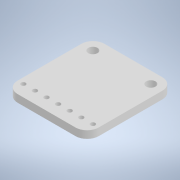
# Autodesk Inventor part: BMP280 footprint
Saved by Autodesk Inventor 2020 (Build 240168000, 168)
## iProperties
Created: 2020-09-26
Part Number: BMP280 footprint
Material: Generic
Document SubType Name: Modeling
Designer: mulve
Density: 1 g/cm^3
Appearance: Default
Author: mulve
Autodesk Inventor part; units mm, degrees
ref_plane "YZ Plane" through (0, 0, 0) normal (1, 0, 0) x (0, 1, 0)
ref_plane "XZ Plane" through (0, 0, 0) normal (0, 1, 0) x (-1, 0, 0)
ref_plane "XY Plane" through (0, 0, 0) normal (0, 0, 1) x (1, 0, 0)
sketch "Sketch1" plane through (0, 0, 0) normal (0, 1, 0) x (-1, 0, 0)
  line L0 (-2.54, 0) -> (-15.24, 0)
  line L1 (-17.78, -2.54) -> (-17.78, -16.51)
  line L2 (-15.24, -19.05) -> (-2.54, -19.05)
  line L3 (0, -16.51) -> (0, -2.54)
  arc A0 (-2.54, -19.05) -> (0, -16.51) centre (-2.54, -16.51) ccw
  arc A1 (-17.78, -16.51) -> (-15.24, -19.05) centre (-15.24, -16.51) ccw
  arc A2 (0, -2.54) -> (-2.54, 0) centre (-2.54, -2.54) ccw
  arc A3 (-15.24, 0) -> (-17.78, -2.54) centre (-15.24, -2.54) ccw
  circle A4 centre (-2.54, -16.51) radius 1.016
  circle A5 centre (-15.24, -16.51) radius 1.016
  line L4 (0, -2.54) -> (-17.78, -2.54) construction
  circle A6 centre (-1.27, -2.54) radius 0.508
  circle A7 centre (-3.81, -2.54) radius 0.508
  circle A8 centre (-6.35, -2.54) radius 0.508
  circle A9 centre (-8.89, -2.54) radius 0.508
  circle A10 centre (-11.43, -2.54) radius 0.508
  circle A11 centre (-13.97, -2.54) radius 0.508
  circle A12 centre (-16.51, -2.54) radius 0.508
  point P0 (0, 0)
  point P1 (-17.78, -19.05)
  point P2 (-17.78, 0)
  point P3 (0, -19.05)
  dimension "d0" = 17.78
  dimension "d1" = 19.05
  dimension "d2" = 2.54
  dimension "d3" = 2.032
  dimension "d6" = 2.54
  dimension "d11" = 1.27
  dimension "d12" = 1.27
  dimension "d13" = 1.016
  dimension "d16" = 2.54
  constraints: 13 centre point, 10 end point, 9 point on line, 8 point on circle, 8 tangent, 4 equal radius, 4 horizontal, 2 coincident, 2 parallel, 1 perpendicular, 18 other
  measures "d0" distance of point (-17.78, -19.05) point (0, -19.05)
  measures "d1" distance of point (-17.78, 0) point (-17.78, -19.05)
  measures "d2" radius of A0
  measures "d3" diameter of A4
  measures "d6" distance of point (-1.27, -2.54) point (-3.81, -2.54)
  measures "d11" distance from line of L1 point (-16.51, -2.54)
  measures "d12" distance from line of L3 point (-1.27, -2.54)
  measures "d13" diameter of A6
  measures "d16" distance of A6.centre A7.centre
extrude "Extrusion1" add sketch "Sketch1" along normal blind 1.65
equation "\"d11\" = d12"
body "Solid1"
